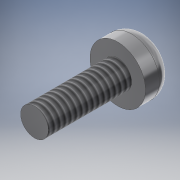
# Autodesk Inventor part: 2x6mmScrew
Saved by Autodesk Inventor 2017 (Build 210142000, 142)
## iProperties
Created: 2019-03-25
Part Number: 2x6mmScrew
Material: Generic
Document SubType Name: Modeling
Designer: cresswnd
Density: 1 g/cm^3
Appearance: Aluminum - Polished
Author: cresswnd
Autodesk Inventor part; units mm, degrees
ref_plane "YZ Plane" through (0, 0, 0) normal (1, 0, 0) x (0, 1, 0)
ref_plane "XZ Plane" through (0, 0, 0) normal (0, 1, 0) x (-1, 0, 0)
ref_plane "XY Plane" through (0, 0, 0) normal (0, 0, 1) x (1, 0, 0)
sketch "Sketch1" plane through (0, 0, 0) normal (0, 1, 0) x (-1, 0, 0)
  circle A0 centre (0, 0) radius 1
  dimension "d0" = 2
  constraints: 1 centre point, 1 coincident
  measures "d0" diameter of A0
extrude "Extrusion1" add sketch "Sketch1" along normal blind 6
sketch "Sketch2" plane through (0, 6, 0) normal (0, 1, 0) x (1, 0, 0)
  circle A0 centre (0, 0) radius 2
  dimension "d3" = 4
  constraints: 1 centre point, 1 coincident
  measures "d3" diameter of A0
extrude "Extrusion2" add sketch "Sketch2" along normal blind 2
sketch "Sketch3" plane through (0, 8, 0) normal (0, 1, 0) x (1, 0, 0)
  circle A0 centre (0, 0) radius 1 construction
  circle A1 centre (0, 0) radius 1 construction
  circle A2 centre (0, 0) radius 1
  line L0 (-0.9996, -0.0278) -> (-0.5239, 0.8518)
  line L1 (-0.5239, 0.8518) -> (0.4758, 0.8796)
  line L2 (0.4758, 0.8796) -> (0.9996, 0.0278)
  line L3 (0.9996, 0.0278) -> (0.5239, -0.8518)
  line L4 (0.5239, -0.8518) -> (-0.4758, -0.8796)
  line L5 (-0.4758, -0.8796) -> (-0.9996, -0.0278)
  dimension "d6" = 2
  constraints: 12 end point, 3 coincident, 19 other
extrude "Extrusion3" cut sketch "Sketch3" against normal blind 1 contours L3 L4 L5 L0 L1 L2
fillet "Fillet1" radius 1 1 edges at (-2, 8, 0)
thread "Thread1" size "M2x0.4" class "6g" standard "ANSI Metric M Profile" full length
body "Solid1"
